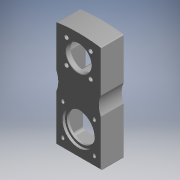
# Autodesk Inventor part: 2607475 EAMM-U-70-D40-60P-96---(UT)
Saved by Autodesk Inventor 2017.3 (Build 213256000, 256)
## iProperties
Part Number: 2607475 EAMM-U-70-D40-60P-96---(UT)
Material: Generic
Catalog Web Link: www.cadenas.de
Description: EAMM-U---(UT)-parallel kit
Vendor: FESTO
Document SubType Name: Modeling
Designer: partserver
Manufacturer: FESTO
Mass: 192.233 g
Surface Area: 562.674 cm^2
Volume: 192.233 cm^3
Density: 1 g/cm^3
Appearance: PSOLRGB-192-192-192
Category: PARTsolutions
Company: FESTO
Title: 2607475 EAMM-U-70-D40-60P-96---(UT)
Author: Cadenas PARTsolutions
Comments: parallel kit
PSOL_IDENT_0: {$CADENAS_DATA\23d-libs\festo\parts\e\eamm\parts\eamm_u_ut.prj},218 {VTYP=3D},{NB=2607475 EAMM-U-70-
PSOL_IDENT_1: D40-60P-96---(UT)},{LINA=2607475 EAMM-U-70-D40-60P-96---(UT)},{NN=EAMM-U---(UT)},{DATE=08.03.2021 13
PSOL_IDENT_2: :38:17},{GEOMDATE=08.03.2021 13:37:58},{VERSION=},{LINEID=860},{WBVAR=},{WBNUMERIC=}  {NB=2607475 EA
PSOL_IDENT_3: MM-U-70-D40-60P-96---(UT)},{LINA=2607475 EAMM-U-70-D40-60P-96---(UT)},{KT=DUMMY},{TNR=2607475},{TYP=
PSOL_IDENT_4: EAMM-U-70-D40-60P-96},{VERS=6},{VERS2=60P},{VERS3=D40},{W1=38.000},{W2=38.000},{H0=96.000},{H5=34.50
PSOL_IDENT_5: 0},{H7=173.500},{H8=48.000},{H10=100.500},{H12=0.000},{L1=36.000},{L4=8.000},{L4A=0.000},{L5=0.000},
PSOL_IDENT_6: {L6=0.000},{D4=0.000},{T2=0.000},{T3=32.600},{T4=0.000},{SAX=24.748737},{SAY=24.748737},{H1=32.500},
PSOL_IDENT_7: {ANZ=4},{DV3=0.000},{DV2=0.000},{DV4=0.000},{DV5=0.000},{DV6=0.000},{TV2=0.000},{LV2=0.000},{DM1=0.0
PSOL_IDENT_8: 00},{DM2=0.000},{TM2=0.000},{LM1=0.000},{DM3=0.000},{DM4=0.000},{LM4=0.000},{RM4=0.000},{DM5=0.000},
PSOL_IDENT_9: {LE1=0.000},{TV4=0.000},{TM3=0.000},{VR=0},{VRS=0},{T1=0.000}
NB: 2607475 EAMM-U-70-D40-60P-96---(UT)
NN: EAMM-U---(UT)
NT: parallel kit
NBSYN: $TNR. $TYP.---(UT)
LINA: 2607475 EAMM-U-70-D40-60P-96---(UT)
CATALOG: Festo
TNR: 2607475
TYP: EAMM-U-70-D40-60P-96
VERS: 6
VERS2: 60P
VERS3: D40
W1: 38
W2: 38
H0: 96
H5: 34.5
H7: 173.5
H8: 48
H10: 100.5
H12: 0
L1: 36
L4: 8
L4A: 0
L5: 0
L6: 0
D4: 0
T2: 0
T3: 32.6
T4: 0
H1: 32.5
ANZ: 4
VR: 0
VRS: 0
SUPPLIER: FESTO
ARTICLENO: 2607475 EAMM-U-70-D40-60P-96---(UT)
BOMINFO: 2607475 EAMM-U-70-D40-60P-96---(UT)
CREATOR: CADENAS GmbH
Autodesk Inventor part; units mm, degrees
sketch "Sketch_1" plane through (0, 0, 0) normal (0, 1, 0) x (-1, 0, 0)
  line L0 (35, -76.5086) -> (35, -3.969)
  arc A0 (35, -3.969) -> (33.7199, -2.4852) centre (33.5, -3.969) ccw
  arc A1 (33.7199, -2.4852) -> (-33.7199, -2.4852) centre (0, -230) ccw
  arc A2 (-33.7199, -2.4852) -> (-35, -3.969) centre (-33.5, -3.969) ccw
  line L1 (-35, -3.969) -> (-35, -76.5086)
  arc A3 (-35, -76.5086) -> (-34.8767, -77.1042) centre (-33.5, -76.5086) ccw
  arc A4 (-34.8767, -104.8958) -> (-34.8767, -77.1042) centre (-67, -91) ccw
  arc A5 (-34.8767, -104.8958) -> (-35, -105.4914) centre (-33.5, -105.4914) ccw
  line L2 (-35, -105.4914) -> (-35, -169.531)
  arc A6 (-35, -169.531) -> (-33.7199, -171.0148) centre (-33.5, -169.531) ccw
  arc A7 (-33.7199, -171.0148) -> (33.7199, -171.0148) centre (0, 56.5) ccw
  arc A8 (33.7199, -171.0148) -> (35, -169.531) centre (33.5, -169.531) ccw
  line L3 (35, -169.531) -> (35, -105.4914)
  arc A9 (35, -105.4914) -> (34.8767, -104.8958) centre (33.5, -105.4914) ccw
  arc A10 (34.8767, -77.1042) -> (34.8767, -104.8958) centre (67, -91) ccw
  arc A11 (34.8767, -77.1042) -> (35, -76.5086) centre (33.5, -76.5086) ccw
  constraints: 24 point on circle, 12 centre point, 8 end point
extrude "Extrusion1" add sketch "Sketch_1" along normal blind 36
sketch "Sketch_2" plane through (0, 0, 0) normal (1, 0, 0) x (0, 1, 0)
  line L0 (5, 0) -> (0, 0)
  line L1 (0, 0) -> (0, -5)
  line L2 (0, -5) -> (5, 0)
  constraints: 6 end point
extrude "Extrusion2" cut sketch "Sketch_2" along normal mid plane 86
sketch "Sketch3" plane through (0, 36, 0) normal (0, 1, 0) x (1, 0, 0)
  point P0 (0, 104.5)
hole "Hole1" at (0, 36, -104.5) direction (0, -1, 0) diameter 6.647 depth 30 tip angle 120 countersink diameter 8 countersink angle 90 thread size "M8x1.25" class "6H" standard "ISO Metric profile"
sketch "Sketch4" plane through (0, 36, 0) normal (0, 1, 0) x (1, 0, 0)
  point P0 (0, 77.5)
hole "Hole2" at (0, 36, -77.5) direction (0, -1, 0) diameter 6.647 depth 30 tip angle 120 countersink diameter 8 countersink angle 90 thread size "M8x1.25" class "6H" standard "ISO Metric profile"
sketch "Sketch5" plane through (0, 36, 0) normal (0, 1, 0) x (1, 0, 0)
  point P0 (-29, 149)
hole "Hole3" at (-29, 36, -149) direction (0, -1, 0) diameter 4.134 depth 18 tip angle 120 countersink diameter 5 countersink angle 90 thread size "M5x0.8" class "6H" standard "ISO Metric profile"
sketch "Sketch6" plane through (0, 36, 0) normal (0, 1, 0) x (1, 0, 0)
  point P0 (-29, 106.5)
hole "Hole4" at (-29, 36, -106.5) direction (0, -1, 0) diameter 4.134 depth 18 tip angle 120 countersink diameter 5 countersink angle 90 thread size "M5x0.8" class "6H" standard "ISO Metric profile"
sketch "Sketch7" plane through (0, 36, 0) normal (0, 1, 0) x (1, 0, 0)
  point P0 (29, 149)
hole "Hole5" at (29, 36, -149) direction (0, -1, 0) diameter 4.134 depth 18 tip angle 120 countersink diameter 5 countersink angle 90 thread size "M5x0.8" class "6H" standard "ISO Metric profile"
sketch "Sketch8" plane through (0, 36, 0) normal (0, 1, 0) x (1, 0, 0)
  point P0 (29, 106.5)
hole "Hole6" at (29, 36, -106.5) direction (0, -1, 0) diameter 4.134 depth 18 tip angle 120 countersink diameter 5 countersink angle 90 thread size "M5x0.8" class "6H" standard "ISO Metric profile"
sketch "Sketch9" plane through (0, 36, 0) normal (0, 1, 0) x (1, 0, 0)
  point P0 (0, 6)
hole "Hole7" at (0, 36, -6) direction (0, -1, 0) diameter 4.134 depth 18 tip angle 120 countersink diameter 5 countersink angle 90 thread size "M5x0.8" class "6H" standard "ISO Metric profile"
sketch "Sketch10" plane through (0, 0, 0) normal (0, -1, 0) x (1, 0, 0)
  point P0 (0, -139)
hole "Hole8" at (0, 0, -139) direction (0, 1, 0) diameter 40 depth 36 countersink diameter 41.2 countersink angle 90
sketch "Sketch11" plane through (0, 36, 0) normal (0, 1, 0) x (1, 0, 0)
  point P0 (19, 120)
hole "Hole9" at (19, 36, -120) direction (0, -1, 0) diameter 6.6 depth 36 counterbore diameter 11 counterbore depth 32.5
sketch "Sketch12" plane through (0, 36, 0) normal (0, 1, 0) x (1, 0, 0)
  point P0 (19, 158)
hole "Hole10" at (19, 36, -158) direction (0, -1, 0) diameter 6.6 depth 36 counterbore diameter 11 counterbore depth 32.5
sketch "Sketch13" plane through (0, 36, 0) normal (0, 1, 0) x (1, 0, 0)
  point P0 (-19, 120)
hole "Hole11" at (-19, 36, -120) direction (0, -1, 0) diameter 6.6 depth 36 counterbore diameter 11 counterbore depth 32.5
sketch "Sketch14" plane through (0, 36, 0) normal (0, 1, 0) x (1, 0, 0)
  point P0 (-19, 158)
hole "Hole12" at (-19, 36, -158) direction (0, -1, 0) diameter 6.6 depth 36 counterbore diameter 11 counterbore depth 32.5
sketch "Sketch_59" plane through (0, 36, 0) normal (0, 1, 0) x (1, 0, 0)
  arc A0 (20.9987, 13.2513) -> (23.9987, 10.2513) centre (23.9987, 13.2513) ccw
  line L0 (23.9987, 10.2513) -> (25.4987, 10.2513)
  arc A1 (25.4987, 10.2513) -> (28.4987, 13.2513) centre (25.4987, 13.2513) ccw
  line L1 (28.4987, 13.2513) -> (28.4987, 23.2513)
  arc A2 (28.4987, 23.2513) -> (25.4987, 26.2513) centre (25.4987, 23.2513) ccw
  line L2 (25.4987, 26.2513) -> (23.9987, 26.2513)
  arc A3 (23.9987, 26.2513) -> (20.9987, 23.2513) centre (23.9987, 23.2513) ccw
  line L3 (20.9987, 23.2513) -> (20.9987, 13.2513)
  constraints: 8 end point, 8 point on circle, 4 centre point
extrude "Extrusion3" cut sketch "Sketch_59" against normal blind 32.6
sketch "Sketch_60" plane through (0, 36, 0) normal (0, 1, 0) x (1, 0, 0)
  arc A0 (20.9987, 62.7487) -> (23.9987, 59.7487) centre (23.9987, 62.7487) ccw
  line L0 (23.9987, 59.7487) -> (25.4987, 59.7487)
  arc A1 (25.4987, 59.7487) -> (28.4987, 62.7487) centre (25.4987, 62.7487) ccw
  line L1 (28.4987, 62.7487) -> (28.4987, 72.7487)
  arc A2 (28.4987, 72.7487) -> (25.4987, 75.7487) centre (25.4987, 72.7487) ccw
  line L2 (25.4987, 75.7487) -> (23.9987, 75.7487)
  arc A3 (23.9987, 75.7487) -> (20.9987, 72.7487) centre (23.9987, 72.7487) ccw
  line L3 (20.9987, 72.7487) -> (20.9987, 62.7487)
  constraints: 8 end point, 8 point on circle, 4 centre point
extrude "Extrusion4" cut sketch "Sketch_60" against normal blind 32.6
sketch "Sketch_61" plane through (0, 36, 0) normal (0, 1, 0) x (1, 0, 0)
  arc A0 (-28.4987, 62.7487) -> (-25.4987, 59.7487) centre (-25.4987, 62.7487) ccw
  line L0 (-25.4987, 59.7487) -> (-23.9987, 59.7487)
  arc A1 (-23.9987, 59.7487) -> (-20.9987, 62.7487) centre (-23.9987, 62.7487) ccw
  line L1 (-20.9987, 62.7487) -> (-20.9987, 72.7487)
  arc A2 (-20.9987, 72.7487) -> (-23.9987, 75.7487) centre (-23.9987, 72.7487) ccw
  line L2 (-23.9987, 75.7487) -> (-25.4987, 75.7487)
  arc A3 (-25.4987, 75.7487) -> (-28.4987, 72.7487) centre (-25.4987, 72.7487) ccw
  line L3 (-28.4987, 72.7487) -> (-28.4987, 62.7487)
  constraints: 8 end point, 8 point on circle, 4 centre point
extrude "Extrusion5" cut sketch "Sketch_61" against normal blind 32.6
sketch "Sketch_62" plane through (0, 36, 0) normal (0, 1, 0) x (1, 0, 0)
  arc A0 (-28.4987, 13.2513) -> (-25.4987, 10.2513) centre (-25.4987, 13.2513) ccw
  line L0 (-25.4987, 10.2513) -> (-23.9987, 10.2513)
  arc A1 (-23.9987, 10.2513) -> (-20.9987, 13.2513) centre (-23.9987, 13.2513) ccw
  line L1 (-20.9987, 13.2513) -> (-20.9987, 23.2513)
  arc A2 (-20.9987, 23.2513) -> (-23.9987, 26.2513) centre (-23.9987, 23.2513) ccw
  line L2 (-23.9987, 26.2513) -> (-25.4987, 26.2513)
  arc A3 (-25.4987, 26.2513) -> (-28.4987, 23.2513) centre (-25.4987, 23.2513) ccw
  line L3 (-28.4987, 23.2513) -> (-28.4987, 13.2513)
  constraints: 8 end point, 8 point on circle, 4 centre point
extrude "Extrusion6" cut sketch "Sketch_62" against normal blind 32.6
sketch "Sketch_64" plane through (0, 36, 0) normal (0, 1, 0) x (1, 0, 0)
  arc A0 (22.5987, 17.2513) -> (26.8987, 17.2513) centre (24.7487, 17.2513) ccw
  line L0 (26.8987, 17.2513) -> (26.8987, 19.2513)
  arc A1 (26.8987, 19.2513) -> (22.5987, 19.2513) centre (24.7487, 19.2513) ccw
  line L1 (22.5987, 19.2513) -> (22.5987, 17.2513)
  constraints: 4 end point, 4 point on circle, 2 centre point
extrude "Extrusion7" cut sketch "Sketch_64" against normal blind 36
sketch "Sketch_65" plane through (0, 36, 0) normal (0, 1, 0) x (1, 0, 0)
  arc A0 (22.5987, 66.7487) -> (26.8987, 66.7487) centre (24.7487, 66.7487) ccw
  line L0 (26.8987, 66.7487) -> (26.8987, 68.7487)
  arc A1 (26.8987, 68.7487) -> (22.5987, 68.7487) centre (24.7487, 68.7487) ccw
  line L1 (22.5987, 68.7487) -> (22.5987, 66.7487)
  constraints: 4 end point, 4 point on circle, 2 centre point
extrude "Extrusion8" cut sketch "Sketch_65" against normal blind 36
sketch "Sketch_66" plane through (0, 36, 0) normal (0, 1, 0) x (1, 0, 0)
  arc A0 (-26.8987, 66.7487) -> (-22.5987, 66.7487) centre (-24.7487, 66.7487) ccw
  line L0 (-22.5987, 66.7487) -> (-22.5987, 68.7487)
  arc A1 (-22.5987, 68.7487) -> (-26.8987, 68.7487) centre (-24.7487, 68.7487) ccw
  line L1 (-26.8987, 68.7487) -> (-26.8987, 66.7487)
  constraints: 4 end point, 4 point on circle, 2 centre point
extrude "Extrusion9" cut sketch "Sketch_66" against normal blind 36
sketch "Sketch_78" plane through (0, 36, 0) normal (0, 1, 0) x (1, 0, 0)
  arc A0 (-26.8987, 17.2513) -> (-22.5987, 17.2513) centre (-24.7487, 17.2513) ccw
  line L0 (-22.5987, 17.2513) -> (-22.5987, 19.2513)
  arc A1 (-22.5987, 19.2513) -> (-26.8987, 19.2513) centre (-24.7487, 19.2513) ccw
  line L1 (-26.8987, 19.2513) -> (-26.8987, 17.2513)
  constraints: 4 end point, 4 point on circle, 2 centre point
extrude "Extrusion10" cut sketch "Sketch_78" against normal blind 36
sketch "Sketch_29" plane through (0, 0, 0) normal (0, 1, 0) x (-1, 0, 0)
  arc A0 (25.25, -42) -> (-25.25, -42) centre (0, -42) ccw
  line L0 (-25.25, -42) -> (-25.25, -44)
  arc A1 (-25.25, -44) -> (25.25, -44) centre (0, -44) ccw
  line L1 (25.25, -44) -> (25.25, -42)
  constraints: 4 end point, 4 point on circle, 2 centre point
extrude "Extrusion11" cut sketch "Sketch_29" along normal blind 4
sketch "Sketch_30" plane through (0, 0, 0) normal (1, 0, 0) x (0, 1, 0)
  line L0 (0, -43) -> (36, -43)
  line L1 (36, -43) -> (36, -65.5)
  line L2 (36, -65.5) -> (0, -65.5)
  line L3 (0, -65.5) -> (0, -43)
  line L4 (0, -43) -> (36, -43)
  constraints: 10 end point
revolve "Revolution1" cut sketch "Sketch_30" angle 360 about axis through (0, 0, -43) along (0, -1, 0)
sketch "Sketch_82" plane through (0, 36, 0) normal (0, 1, 0) x (1, 0, 0)
  arc A0 (-28.9987, 13.7513) -> (-24.9987, 9.7513) centre (-24.9987, 13.7513) ccw
  line L0 (-24.9987, 9.7513) -> (24.9987, 9.7513)
  arc A1 (24.9987, 9.7513) -> (28.9987, 13.7513) centre (24.9987, 13.7513) ccw
  line L1 (28.9987, 13.7513) -> (28.9987, 72.2487)
  arc A2 (28.9987, 72.2487) -> (26.9994, 75.7125) centre (24.9987, 72.2487) ccw
  arc A3 (25, 79.1762) -> (26.9994, 75.7125) centre (29, 79.1762) ccw
  line L2 (25, 79.1762) -> (25, 131.8586)
  arc A4 (25, 131.8586) -> (23.2467, 150.6444) centre (0, 139) ccw
  arc A5 (23.5635, 154.7543) -> (23.2467, 150.6444) centre (26.8231, 152.4359) ccw
  arc A6 (23.5635, 154.7543) -> (15.7543, 162.5635) centre (19, 158) ccw
  arc A7 (11.6444, 162.2467) -> (15.7543, 162.5635) centre (13.4359, 165.8231) ccw
  arc A8 (11.6444, 162.2467) -> (-11.6444, 162.2467) centre (0, 139) ccw
  arc A9 (-15.7543, 162.5635) -> (-11.6444, 162.2467) centre (-13.4359, 165.8231) ccw
  arc A10 (-15.7543, 162.5635) -> (-23.5635, 154.7543) centre (-19, 158) ccw
  arc A11 (-23.2467, 150.6444) -> (-23.5635, 154.7543) centre (-26.8231, 152.4359) ccw
  arc A12 (-23.2467, 150.6444) -> (-25, 131.8586) centre (0, 139) ccw
  line L3 (-25, 131.8586) -> (-25, 79.1762)
  arc A13 (-26.9994, 75.7125) -> (-25, 79.1762) centre (-29, 79.1762) ccw
  arc A14 (-26.9994, 75.7125) -> (-28.9987, 72.2487) centre (-24.9987, 72.2487) ccw
  line L4 (-28.9987, 72.2487) -> (-28.9987, 13.7513)
  line L5 (-11.5, 109) -> (-11.5, 73)
  arc A15 (-11.5, 73) -> (-7.5, 69) centre (-7.5, 73) ccw
  line L6 (-7.5, 69) -> (7.5, 69)
  arc A16 (7.5, 69) -> (11.5, 73) centre (7.5, 73) ccw
  line L7 (11.5, 73) -> (11.5, 109)
  arc A17 (11.5, 109) -> (7.5, 113) centre (7.5, 109) ccw
  line L8 (7.5, 113) -> (-7.5, 113)
  arc A18 (-7.5, 113) -> (-11.5, 109) centre (-7.5, 109) ccw
  constraints: 38 point on circle, 19 centre point, 18 end point
extrude "Extrusion12" cut sketch "Sketch_82" against normal blind 28.5
ref_plane "ANBAU_XY" through (0, 0, -139) normal (0, 1, 0) x (1, 0, 0)
ref_plane "ANBAU_YZ" through (0, 0, -139) normal (1, 0, 0) x (0, 0, -1)
ref_plane "ANBAU_ZX" through (0, 0, -139) normal (0, 0, -1) x (0, 1, 0)
ref_plane "AS_1_XY" through (19, 3.5, -120) normal (0, 1, 0) x (1, 0, 0)
ref_plane "AS_1_YZ" through (19, 3.5, -120) normal (1, 0, 0) x (0, 0, -1)
ref_plane "AS_1_ZX" through (19, 3.5, -120) normal (0, 0, -1) x (0, 1, 0)
ref_plane "AS_2_XY" through (19, 3.5, -158) normal (0, 1, 0) x (1, 0, 0)
ref_plane "AS_2_YZ" through (19, 3.5, -158) normal (1, 0, 0) x (0, 0, -1)
ref_plane "AS_2_ZX" through (19, 3.5, -158) normal (0, 0, -1) x (0, 1, 0)
ref_plane "AS_3_XY" through (-19, 3.5, -120) normal (0, 1, 0) x (1, 0, 0)
ref_plane "AS_3_YZ" through (-19, 3.5, -120) normal (1, 0, 0) x (0, 0, -1)
ref_plane "AS_3_ZX" through (-19, 3.5, -120) normal (0, 0, -1) x (0, 1, 0)
ref_plane "AS_4_XY" through (-19, 3.5, -158) normal (0, 1, 0) x (1, 0, 0)
ref_plane "AS_4_YZ" through (-19, 3.5, -158) normal (1, 0, 0) x (0, 0, -1)
ref_plane "AS_4_ZX" through (-19, 3.5, -158) normal (0, 0, -1) x (0, 1, 0)
ref_plane "DM_XY" through (0, 0, -43) normal (0, 1, 0) x (1, 0, 0)
ref_plane "DM_YZ" through (0, 0, -43) normal (1, 0, 0) x (0, 0, -1)
ref_plane "DM_ZX" through (0, 0, -43) normal (0, 0, -1) x (0, 1, 0)
ref_plane "MS_1_XY" through (24.7487, -8, -18.2513) normal (0, 1, 0) x (1, 0, 0)
ref_plane "MS_1_YZ" through (24.7487, -8, -18.2513) normal (1, 0, 0) x (0, 0, -1)
ref_plane "MS_1_ZX" through (24.7487, -8, -18.2513) normal (0, 0, -1) x (0, 1, 0)
ref_plane "MS_2_XY" through (24.7487, -8, -67.7487) normal (0, 1, 0) x (1, 0, 0)
ref_plane "MS_2_YZ" through (24.7487, -8, -67.7487) normal (1, 0, 0) x (0, 0, -1)
ref_plane "MS_2_ZX" through (24.7487, -8, -67.7487) normal (0, 0, -1) x (0, 1, 0)
ref_plane "MS_3_XY" through (-24.7487, -8, -67.7487) normal (0, 1, 0) x (1, 0, 0)
ref_plane "MS_3_YZ" through (-24.7487, -8, -67.7487) normal (1, 0, 0) x (0, 0, -1)
ref_plane "MS_3_ZX" through (-24.7487, -8, -67.7487) normal (0, 0, -1) x (0, 1, 0)
ref_plane "MS_4_XY" through (-24.7487, -8, -18.2513) normal (0, 1, 0) x (1, 0, 0)
ref_plane "MS_4_YZ" through (-24.7487, -8, -18.2513) normal (1, 0, 0) x (0, 0, -1)
ref_plane "MS_4_ZX" through (-24.7487, -8, -18.2513) normal (0, 0, -1) x (0, 1, 0)
ref_plane "OBERTEIL_XY" through (0, 36, -139) normal (0, 1, 0) x (1, 0, 0)
ref_plane "OBERTEIL_YZ" through (0, 36, -139) normal (1, 0, 0) x (0, 0, -1)
ref_plane "OBERTEIL_ZX" through (0, 36, -139) normal (0, 0, -1) x (0, 1, 0)
ref_plane "VM_1_XY" through (24.7487, 3.4, -18.2513) normal (0, 1, 0) x (1, 0, 0)
ref_plane "VM_1_YZ" through (24.7487, 3.4, -18.2513) normal (1, 0, 0) x (0, 0, -1)
ref_plane "VM_1_ZX" through (24.7487, 3.4, -18.2513) normal (0, 0, -1) x (0, 1, 0)
ref_plane "VM_2_XY" through (24.7487, 3.4, -67.7487) normal (0, 1, 0) x (1, 0, 0)
ref_plane "VM_2_YZ" through (24.7487, 3.4, -67.7487) normal (1, 0, 0) x (0, 0, -1)
ref_plane "VM_2_ZX" through (24.7487, 3.4, -67.7487) normal (0, 0, -1) x (0, 1, 0)
ref_plane "VM_3_XY" through (-24.7487, 3.4, -67.7487) normal (0, 1, 0) x (1, 0, 0)
ref_plane "VM_3_YZ" through (-24.7487, 3.4, -67.7487) normal (1, 0, 0) x (0, 0, -1)
ref_plane "VM_3_ZX" through (-24.7487, 3.4, -67.7487) normal (0, 0, -1) x (0, 1, 0)
ref_plane "VM_4_XY" through (-24.7487, 3.4, -18.2513) normal (0, 1, 0) x (1, 0, 0)
ref_plane "VM_4_YZ" through (-24.7487, 3.4, -18.2513) normal (1, 0, 0) x (0, 0, -1)
ref_plane "VM_4_ZX" through (-24.7487, 3.4, -18.2513) normal (0, 0, -1) x (0, 1, 0)
ref_plane "VM_1_1_XY" through (24.7487, 3.4, -18.2513) normal (0, 1, 0) x (1, 0, 0)
ref_plane "VM_1_1_YZ" through (24.7487, 3.4, -18.2513) normal (1, 0, 0) x (0, 0, -1)
ref_plane "VM_1_1_ZX" through (24.7487, 3.4, -18.2513) normal (0, 0, -1) x (0, 1, 0)
ref_plane "VM_1_2_XY" through (24.7487, 3.4, -67.7487) normal (0, 1, 0) x (1, 0, 0)
ref_plane "VM_1_2_YZ" through (24.7487, 3.4, -67.7487) normal (1, 0, 0) x (0, 0, -1)
ref_plane "VM_1_2_ZX" through (24.7487, 3.4, -67.7487) normal (0, 0, -1) x (0, 1, 0)
ref_plane "VM_1_3_XY" through (-24.7487, 3.4, -67.7487) normal (0, 1, 0) x (1, 0, 0)
ref_plane "VM_1_3_YZ" through (-24.7487, 3.4, -67.7487) normal (1, 0, 0) x (0, 0, -1)
ref_plane "VM_1_3_ZX" through (-24.7487, 3.4, -67.7487) normal (0, 0, -1) x (0, 1, 0)
ref_plane "VM_1_4_XY" through (-24.7487, 3.4, -18.2513) normal (0, 1, 0) x (1, 0, 0)
ref_plane "VM_1_4_YZ" through (-24.7487, 3.4, -18.2513) normal (1, 0, 0) x (0, 0, -1)
ref_plane "VM_1_4_ZX" through (-24.7487, 3.4, -18.2513) normal (0, 0, -1) x (0, 1, 0)
ref_plane "ZR_XY" through (0, 0, -139) normal (0, 1, 0) x (1, 0, 0)
ref_plane "ZR_YZ" through (0, 0, -139) normal (1, 0, 0) x (0, 0, -1)
ref_plane "ZR_ZX" through (0, 0, -139) normal (0, 0, -1) x (0, 1, 0)
ref_plane "to_sleeve_1_XY" through (24.7487, -8, -18.2513) normal (0, 1, 0) x (1, 0, 0)
ref_plane "to_sleeve_1_YZ" through (24.7487, -8, -18.2513) normal (1, 0, 0) x (0, 0, -1)
ref_plane "to_sleeve_1_ZX" through (24.7487, -8, -18.2513) normal (0, 0, -1) x (0, 1, 0)
ref_plane "to_sleeve_2_XY" through (24.7487, -8, -67.7487) normal (0, 1, 0) x (1, 0, 0)
ref_plane "to_sleeve_2_YZ" through (24.7487, -8, -67.7487) normal (1, 0, 0) x (0, 0, -1)
ref_plane "to_sleeve_2_ZX" through (24.7487, -8, -67.7487) normal (0, 0, -1) x (0, 1, 0)
ref_plane "to_sleeve_3_XY" through (-24.7487, -8, -67.7487) normal (0, 1, 0) x (1, 0, 0)
ref_plane "to_sleeve_3_YZ" through (-24.7487, -8, -67.7487) normal (1, 0, 0) x (0, 0, -1)
ref_plane "to_sleeve_3_ZX" through (-24.7487, -8, -67.7487) normal (0, 0, -1) x (0, 1, 0)
ref_plane "to_sleeve_4_XY" through (-24.7487, -8, -18.2513) normal (0, 1, 0) x (1, 0, 0)
ref_plane "to_sleeve_4_YZ" through (-24.7487, -8, -18.2513) normal (1, 0, 0) x (0, 0, -1)
ref_plane "to_sleeve_4_ZX" through (-24.7487, -8, -18.2513) normal (0, 0, -1) x (0, 1, 0)
body "Solid1"
